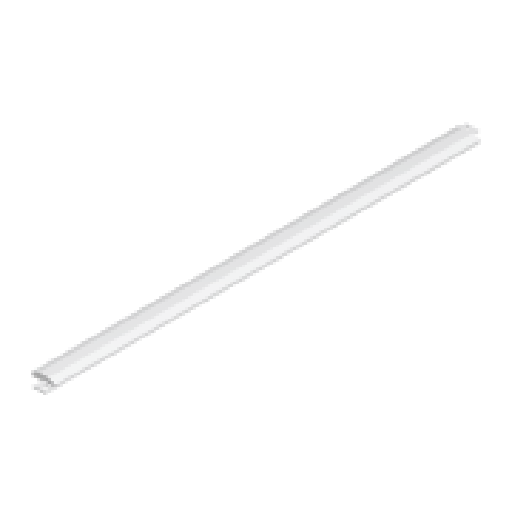
# Autodesk Inventor part: ZLF Alumiline 310
Saved by Autodesk Inventor 2023.2 (Build 272271000, 271)
## iProperties
Created: 2023-02-05
Part Number: ZLF Alumiline 310
Material: Aluminum 6061
Document SubType Name: Modeling
Designer: remop
Density: 2.7 g/cm^3
Appearance: Aluminum - Flat
Author: remop
Autodesk Inventor part; units mm, degrees
ref_plane "YZ Plane" through (0, 0, 0) normal (1, 0, 0) x (0, 1, 0)
ref_plane "XZ Plane" through (0, 0, 0) normal (0, 1, 0) x (-1, 0, 0)
ref_plane "XY Plane" through (0, 0, 0) normal (0, 0, 1) x (1, 0, 0)
sketch "Sketch1" plane through (0, 0, 0) normal (0, 1, 0) x (-1, 0, 0)
  line L0 (-8.5, -155) -> (8.5, -155)
  line L1 (8.5, -155) -> (8.5, 155)
  line L2 (8.5, 155) -> (-8.5, 155)
  line L3 (-8.5, 155) -> (-8.5, -155)
  line L4 (-8.5, -155) -> (8.5, 155) construction
  line L5 (8.5, -155) -> (-8.5, 155) construction
  point P0 (0, 0)
  dimension "d0" = 310
  dimension "d1" = 17
  constraints: 12 end point, 2 midpoint, 2 parallel, 1 horizontal, 1 perpendicular
  measures "d0" distance of L0.end L1.end
  measures "d1" distance of L1.end L2.end
extrude "Extrusion1" add sketch "Sketch1" along normal blind 4.4
chamfer "Chamfer1" distance 5 distance2 2 1 edges at (8.5, 4.4, 0) measured on face at (2.8333, 4.4, 51.6667)
chamfer "Chamfer2" distance 5 distance2 2 1 edges at (-8.5, 4.4, 0) measured on face at (-4.5, 4.4, 51.6667)
sketch "Sketch2" plane through (0, 0, 0) normal (0, -1, 0) x (1, 0, 0)
  line L0 (-8.5, -155) -> (-8.5, 155) projected
  line L1 (8.5, -155) -> (-8.5, -155) projected
  line L2 (8.5, 155) -> (8.5, -155) projected
  line L3 (-8.5, 155) -> (8.5, 155) projected
  circle A0 centre (-5, -158.5) radius 1.75
  circle A1 centre (5, 158.5) radius 1.75
  line L4 (-8.5, 155) -> (8.5, 155) projected
  line L5 (8.5, 155) -> (8.5, 162)
  line L6 (8.5, 162) -> (-0.5, 162)
  line L7 (-0.5, 162) -> (-0.5, 155)
  line L8 (-8.5, -155) -> (-8.5, 155) projected
  line L9 (-8.5, -155) -> (-8.5, -162)
  line L10 (-8.5, -162) -> (0.5, -162)
  line L11 (0.5, -162) -> (0.5, -155)
  line L12 (8.5, -155) -> (-8.5, -155) projected
  point P0 (0, 0)
  dimension "d10" = 3.5
  dimension "d11" = 3.5
  dimension "d12" = 3.5
  dimension "d13" = 3.5
  dimension "d14" = 3.5
  dimension "d15" = 9
  dimension "d16" = 7
  constraints: 12 end point, 4 perpendicular, 2 centre point, 2 parallel, 2 point on line, 2 vertical, 1 equal radius
  measures "d10" distance from line of L3 A1.centre
  measures "d11" distance from line of L1 A0.centre
  measures "d12" diameter of A0
  measures "d13" distance from line of A1.centre L2
  measures "d14" distance from line of L0 A0.centre
  measures "d15" distance of L9.end L10.end
  measures "d16" distance of L0.start L9.end
extrude "Extrusion2" add sketch "Sketch2" against normal blind 1 contours L1 L11 L10 L9 | L7 L6 L5 L3
sketch "Sketch3" plane through (0, 0, 0) normal (0, -1, 0) x (1, 0, 0)
  circle A0 centre (5, 158.5) radius 1.75 projected
  circle A1 centre (-5, -158.5) radius 1.75 projected
  line L0 (-8.5, -162) -> (-8.5, 155) projected
  line L1 (-8.5, -162) -> (0.5, -162) projected
  line L2 (0.5, -162) -> (0.5, -155) projected
  line L3 (8.5, -155) -> (0.5, -155) projected
  line L4 (8.5, -155) -> (8.5, 162) projected
  line L5 (8.5, 162) -> (-0.5, 162) projected
  line L6 (-0.5, 162) -> (-0.5, 155) projected
  line L7 (-8.5, 155) -> (-0.5, 155) projected
  line L8 (5.5, -152) -> (-5.5, -152)
  line L9 (-5.5, -152) -> (-5.5, 152)
  line L10 (-5.5, 152) -> (5.5, 152)
  line L11 (5.5, 152) -> (5.5, -152)
  line L12 (8.5, -155) -> (0.5, -155) projected
  point P0 (0, 0)
  point P1 (4.5, -155)
  dimension "d19" = 3
  dimension "d20" = 3
  dimension "d21" = 3
  dimension "d22" = 3
  constraints: 8 end point, 2 parallel, 1 horizontal, 1 midpoint, 1 perpendicular
  measures "d19" distance between parallel lines of L0 L9
  measures "d20" distance between parallel lines of L4 L11
  measures "d21" distance between parallel lines of L7 L10
  measures "d22" distance from line of point (4.5, -155) L8
extrude "Extrusion3" cut sketch "Sketch3" against normal blind 1 contours L8 L9 L10 L11
equation "\"d11\" = d10"
equation "\"d13\" = d10"
equation "\"d14\" = d10"
equation "\"d16\" = 2 * d14"
equation "\"d20\" = d19"
equation "\"d21\" = d19"
equation "\"d22\" = d19"
body "Solid1"
